Autodesk Fusion 360 part; units mm, degrees
(part 2 of 6)
  spline S37 degree 5 poles (-61.6244, -22.3751) (-61.6253, -22.3767) (-61.6305, -22.3859) (-61.6398, -22.4027) (-61.6532, -22.4272) (-61.6708, -22.4593) (-61.6915, -22.4977) (-61.7119, -22.5363) (-61.7322, -22.5749) (-61.7524, -22.6137) (-61.7724, -22.6527) (-61.7922, -22.6917) (-61.8118, -22.7309) (-61.8313, -22.7703) (-61.8506, -22.8097) (-61.8697, -22.8493) (-61.8887, -22.889) (-61.9075, -22.9288) (-61.9262, -22.9687) (-61.9447, -23.0088) (-61.963, -23.049) (-61.9812, -23.0893) (-61.9993, -23.1297) (-62.0172, -23.1702) (-62.035, -23.2108) (-62.0526, -23.2515) (-62.07, -23.2924) (-62.0873, -23.3333) (-62.1045, -23.3744) (-62.1215, -23.4155) (-62.1384, -23.4568) (-62.1551, -23.4982) (-62.1717, -23.5396) (-62.1882, -23.5812) (-62.2045, -23.6228) (-62.2207, -23.6646) (-62.2367, -23.7064) (-62.2526, -23.7484) (-62.2683, -23.7904) (-62.284, -23.8326) (-62.2995, -23.8748) (-62.3148, -23.9171) (-62.33, -23.9595) (-62.3451, -24.0021) (-62.3601, -24.0446) (-62.3749, -24.0873) (-62.3896, -24.1301) (-62.4012, -24.1644) (-62.4099, -24.1901) (-62.4156, -24.2073) (-62.4185, -24.2159) knots 0.354152 0.354152 0.354152 0.354152 0.354152 0.354152 0.357143 0.371429 0.385714 0.4 0.414286 0.428571 0.442857 0.457143 0.471429 0.485714 0.5 0.514286 0.528571 0.542857 0.557143 0.571429 0.585714 0.6 0.614286 0.628571 0.642857 0.657143 0.671429 0.685714 0.7 0.714286 0.728571 0.742857 0.757143 0.771429 0.785714 0.8 0.814286 0.828571 0.842857 0.857143 0.871429 0.885714 0.9 0.914286 0.928571 0.942857 0.957143 0.971429 0.985714 1 1 1 1 1 1
  arc A19 (-62.4185, -24.2159) -> (-61.8912, -24.6937) centre (-40, 0) ccw
  spline S38 degree 5 poles (-61.8912, -24.6937) (-61.8829, -24.69) (-61.8663, -24.6826) (-61.8416, -24.6714) (-61.8086, -24.6564) (-61.7675, -24.6376) (-61.7265, -24.6187) (-61.6855, -24.5996) (-61.6447, -24.5804) (-61.604, -24.5611) (-61.5634, -24.5416) (-61.5229, -24.5221) (-61.4825, -24.5024) (-61.4422, -24.4825) (-61.402, -24.4626) (-61.362, -24.4425) (-61.322, -24.4223) (-61.2822, -24.402) (-61.2424, -24.3815) (-61.2028, -24.3609) (-61.1633, -24.3402) (-61.1239, -24.3193) (-61.0846, -24.2983) (-61.0454, -24.2772) (-61.0064, -24.256) (-60.9675, -24.2346) (-60.9287, -24.213) (-60.89, -24.1914) (-60.8514, -24.1696) (-60.813, -24.1476) (-60.7747, -24.1255) (-60.7365, -24.1033) (-60.6985, -24.081) (-60.6606, -24.0585) (-60.6228, -24.0358) (-60.5852, -24.013) (-60.5477, -23.9901) (-60.5103, -23.967) (-60.4731, -23.9437) (-60.436, -23.9203) (-60.3991, -23.8968) (-60.3623, -23.8731) (-60.3257, -23.8492) (-60.2892, -23.8252) (-60.2529, -23.801) (-60.2167, -23.7767) (-60.1864, -23.756) (-60.1634, -23.7402) (-60.1476, -23.7293) (-60.1389, -23.7233) (-60.1374, -23.7223) knots -1 -1 -1 -1 -1 -1 -0.985714 -0.971429 -0.957143 -0.942857 -0.928571 -0.914286 -0.9 -0.885714 -0.871429 -0.857143 -0.842857 -0.828571 -0.814286 -0.8 -0.785714 -0.771429 -0.757143 -0.742857 -0.728571 -0.714286 -0.7 -0.685714 -0.671429 -0.657143 -0.642857 -0.628571 -0.614286 -0.6 -0.585714 -0.571429 -0.557143 -0.542857 -0.528571 -0.514286 -0.5 -0.485714 -0.471429 -0.457143 -0.442857 -0.428571 -0.414286 -0.4 -0.385714 -0.371429 -0.357143 -0.354152 -0.354152 -0.354152 -0.354152 -0.354152 -0.354152
  spline S39 degree 3 poles (-59.5346, -23.7468) (-59.5849, -23.7055) (-59.6428, -23.6743) (-59.7672, -23.636) (-59.8326, -23.6291) (-59.9404, -23.6389) (-59.9826, -23.6483) (-60.0636, -23.6778) (-60.102, -23.6977) (-60.1374, -23.7223) knots 0 0 0 0 0.019532 0.019532 0.039064 0.039064 0.051994 0.051994 0.064924 0.064924 0.064924 0.064924
  arc A20 (-59.5346, -23.7468) -> (-59.4691, -23.8006) centre (-40, 0) ccw
  spline S40 degree 3 poles (-59.3272, -24.3869) (-59.3012, -24.3272) (-59.2872, -24.263) (-59.2845, -24.1328) (-59.2958, -24.0681) (-59.3348, -23.9672) (-59.3555, -23.9291) (-59.4061, -23.8593) (-59.4358, -23.8278) (-59.4691, -23.8006) knots 0 0 0 0 0.019532 0.019532 0.039064 0.039064 0.051994 0.051994 0.064924 0.064924 0.064924 0.064924
  spline S41 degree 5 poles (-59.3272, -24.3869) (-59.3279, -24.3886) (-59.3321, -24.3982) (-59.3397, -24.4159) (-59.3507, -24.4416) (-59.365, -24.4753) (-59.3818, -24.5155) (-59.3985, -24.5559) (-59.4149, -24.5964) (-59.4311, -24.6369) (-59.4472, -24.6776) (-59.463, -24.7185) (-59.4787, -24.7594) (-59.4943, -24.8004) (-59.5096, -24.8416) (-59.5248, -24.8829) (-59.5398, -24.9242) (-59.5546, -24.9657) (-59.5693, -25.0073) (-59.5838, -25.049) (-59.5981, -25.0907) (-59.6123, -25.1326) (-59.6263, -25.1746) (-59.6401, -25.2167) (-59.6538, -25.2588) (-59.6673, -25.3011) (-59.6807, -25.3435) (-59.6939, -25.3859) (-59.707, -25.4284) (-59.7199, -25.4711) (-59.7326, -25.5138) (-59.7452, -25.5566) (-59.7577, -25.5995) (-59.77, -25.6424) (-59.7821, -25.6855) (-59.7941, -25.7286) (-59.806, -25.7719) (-59.8177, -25.8152) (-59.8292, -25.8586) (-59.8407, -25.902) (-59.8519, -25.9456) (-59.8631, -25.9892) (-59.874, -26.0329) (-59.8849, -26.0767) (-59.8956, -26.1205) (-59.9062, -26.1645) (-59.9166, -26.2085) (-59.9248, -26.2437) (-59.9309, -26.2702) (-59.935, -26.2879) (-59.937, -26.2967) knots 0.354152 0.354152 0.354152 0.354152 0.354152 0.354152 0.357143 0.371429 0.385714 0.4 0.414286 0.428571 0.442857 0.457143 0.471429 0.485714 0.5 0.514286 0.528571 0.542857 0.557143 0.571429 0.585714 0.6 0.614286 0.628571 0.642857 0.657143 0.671429 0.685714 0.7 0.714286 0.728571 0.742857 0.757143 0.771429 0.785714 0.8 0.814286 0.828571 0.842857 0.857143 0.871429 0.885714 0.9 0.914286 0.928571 0.942857 0.957143 0.971429 0.985714 1 1 1 1 1 1
  arc A21 (-59.937, -26.2967) -> (-59.3653, -26.7205) centre (-40, 0) ccw
  spline S42 degree 5 poles (-59.3653, -26.7205) (-59.3575, -26.716) (-59.3417, -26.707) (-59.3182, -26.6934) (-59.2868, -26.6753) (-59.2477, -26.6525) (-59.2088, -26.6297) (-59.1699, -26.6067) (-59.1312, -26.5836) (-59.0926, -26.5604) (-59.0541, -26.537) (-59.0157, -26.5136) (-58.9774, -26.49) (-58.9393, -26.4664) (-58.9012, -26.4426) (-58.8633, -26.4187) (-58.8255, -26.3946) (-58.7879, -26.3705) (-58.7503, -26.3462) (-58.7129, -26.3219) (-58.6756, -26.2974) (-58.6385, -26.2727) (-58.6014, -26.248) (-58.5645, -26.2231) (-58.5277, -26.1982) (-58.4911, -26.173) (-58.4546, -26.1478) (-58.4182, -26.1225) (-58.382, -26.097) (-58.3459, -26.0714) (-58.31, -26.0457) (-58.2741, -26.0198) (-58.2385, -25.9938) (-58.203, -25.9677) (-58.1676, -25.9414) (-58.1324, -25.9151) (-58.0973, -25.8886) (-58.0624, -25.8619) (-58.0276, -25.8351) (-57.993, -25.8082) (-57.9586, -25.7812) (-57.9243, -25.754) (-57.8902, -25.7266) (-57.8562, -25.6992) (-57.8225, -25.6715) (-57.7888, -25.6438) (-57.7607, -25.6203) (-57.7393, -25.6023) (-57.7247, -25.5898) (-57.7167, -25.583) (-57.7153, -25.5818) knots -1 -1 -1 -1 -1 -1 -0.985714 -0.971429 -0.957143 -0.942857 -0.928571 -0.914286 -0.9 -0.885714 -0.871429 -0.857143 -0.842857 -0.828571 -0.814286 -0.8 -0.785714 -0.771429 -0.757143 -0.742857 -0.728571 -0.714286 -0.7 -0.685714 -0.671429 -0.657143 -0.642857 -0.628571 -0.614286 -0.6 -0.585714 -0.571429 -0.557143 -0.542857 -0.528571 -0.514286 -0.5 -0.485714 -0.471429 -0.457143 -0.442857 -0.428571 -0.414286 -0.4 -0.385714 -0.371429 -0.357143 -0.354152 -0.354152 -0.354152 -0.354152 -0.354152 -0.354152
  spline S43 degree 3 poles (-57.113, -25.5472) (-57.1671, -25.511) (-57.2277, -25.4856) (-57.3553, -25.4597) (-57.421, -25.4593) (-57.5273, -25.4796) (-57.5684, -25.4931) (-57.6462, -25.5303) (-57.6825, -25.5539) (-57.7153, -25.5818) knots 0 0 0 0 0.019532 0.019532 0.039064 0.039064 0.051994 0.051994 0.064924 0.064924 0.064924 0.064924
  arc A22 (-57.113, -25.5472) -> (-57.0425, -25.5943) centre (-40, 0) ccw
  spline S44 degree 3 poles (-56.8438, -26.1639) (-56.8238, -26.1019) (-56.8161, -26.0367) (-56.8262, -25.9068) (-56.8438, -25.8435) (-56.8925, -25.7469) (-56.9168, -25.7111) (-56.974, -25.6466) (-57.0066, -25.6181) (-57.0425, -25.5943) knots 0 0 0 0 0.019532 0.019532 0.039064 0.039064 0.051994 0.051994 0.064924 0.064924 0.064924 0.064924
  spline S45 degree 5 poles (-56.8438, -26.1639) (-56.8443, -26.1656) (-56.8476, -26.1756) (-56.8534, -26.1939) (-56.8619, -26.2206) (-56.8728, -26.2556) (-56.8856, -26.2972) (-56.8981, -26.339) (-56.9105, -26.3809) (-56.9227, -26.4229) (-56.9347, -26.465) (-56.9465, -26.5072) (-56.9581, -26.5494) (-56.9695, -26.5918) (-56.9808, -26.6343) (-56.9918, -26.6768) (-57.0027, -26.7194) (-57.0134, -26.7622) (-57.0239, -26.805) (-57.0342, -26.8479) (-57.0444, -26.8909) (-57.0544, -26.9339) (-57.0642, -26.9771) (-57.0739, -27.0203) (-57.0834, -27.0636) (-57.0927, -27.107) (-57.1018, -27.1505) (-57.1108, -27.194) (-57.1196, -27.2376) (-57.1283, -27.2813) (-57.1368, -27.3251) (-57.1452, -27.3689) (-57.1533, -27.4128) (-57.1614, -27.4568) (-57.1692, -27.5008) (-57.177, -27.5449) (-57.1845, -27.5891) (-57.1919, -27.6333) (-57.1992, -27.6777) (-57.2063, -27.722) (-57.2132, -27.7665) (-57.22, -27.811) (-57.2267, -27.8555) (-57.2332, -27.9002) (-57.2395, -27.9449) (-57.2457, -27.9896) (-57.2518, -28.0344) (-57.2565, -28.0703) (-57.26, -28.0973) (-57.2623, -28.1153) (-57.2634, -28.1243) knots 0.354152 0.354152 0.354152 0.354152 0.354152 0.354152 0.357143 0.371429 0.385714 0.4 0.414286 0.428571 0.442857 0.457143 0.471429 0.485714 0.5 0.514286 0.528571 0.542857 0.557143 0.571429 0.585714 0.6 0.614286 0.628571 0.642857 0.657143 0.671429 0.685714 0.7 0.714286 0.728571 0.742857 0.757143 0.771429 0.785714 0.8 0.814286 0.828571 0.842857 0.857143 0.871429 0.885714 0.9 0.914286 0.928571 0.942857 0.957143 0.971429 0.985714 1 1 1 1 1 1
  arc A23 (-57.2634, -28.1243) -> (-56.653, -28.4899) centre (-40, 0) ccw
  spline S46 degree 5 poles (-56.653, -28.4899) (-56.6456, -28.4847) (-56.6309, -28.4742) (-56.6087, -28.4584) (-56.5793, -28.4373) (-56.5427, -28.4108) (-56.5061, -28.3842) (-56.4697, -28.3575) (-56.4334, -28.3308) (-56.3973, -28.3039) (-56.3612, -28.2769) (-56.3253, -28.2498) (-56.2896, -28.2226) (-56.2539, -28.1953) (-56.2184, -28.1679) (-56.183, -28.1404) (-56.1478, -28.1128) (-56.1126, -28.085) (-56.0777, -28.0572) (-56.0428, -28.0293) (-56.0081, -28.0013) (-55.9735, -27.9731) (-55.9391, -27.9449) (-55.9048, -27.9165) (-55.8707, -27.888) (-55.8367, -27.8595) (-55.8028, -27.8308) (-55.7691, -27.802) (-55.7355, -27.7731) (-55.7021, -27.7441) (-55.6689, -27.7149) (-55.6358, -27.6857) (-55.6028, -27.6563) (-55.57, -27.6269) (-55.5374, -27.5973) (-55.5049, -27.5676) (-55.4726, -27.5377) (-55.4405, -27.5078) (-55.4085, -27.4777) (-55.3767, -27.4476) (-55.3451, -27.4173) (-55.3137, -27.3868) (-55.2824, -27.3563) (-55.2513, -27.3256) (-55.2204, -27.2948) (-55.1897, -27.2639) (-55.164, -27.2377) (-55.1445, -27.2177) (-55.1311, -27.2039) (-55.1238, -27.1964) (-55.1225, -27.1951) knots -1 -1 -1 -1 -1 -1 -0.985714 -0.971429 -0.957143 -0.942857 -0.928571 -0.914286 -0.9 -0.885714 -0.871429 -0.857143 -0.842857 -0.828571 -0.814286 -0.8 -0.785714 -0.771429 -0.757143 -0.742857 -0.728571 -0.714286 -0.7 -0.685714 -0.671429 -0.657143 -0.642857 -0.628571 -0.614286 -0.6 -0.585714 -0.571429 -0.557143 -0.542857 -0.528571 -0.514286 -0.5 -0.485714 -0.471429 -0.457143 -0.442857 -0.428571 -0.414286 -0.4 -0.385714 -0.371429 -0.357143 -0.354152 -0.354152 -0.354152 -0.354152 -0.354152 -0.354152
  spline S47 degree 3 poles (-54.5265, -27.1015) (-54.5839, -27.0708) (-54.6467, -27.0515) (-54.7763, -27.0382) (-54.8417, -27.0442) (-54.9455, -27.0749) (-54.9851, -27.0923) (-55.0588, -27.137) (-55.0926, -27.164) (-55.1225, -27.1951) knots 0 0 0 0 0.019532 0.019532 0.039064 0.039064 0.051994 0.051994 0.064924 0.064924 0.064924 0.064924
  arc A24 (-54.5265, -27.1015) -> (-54.4518, -27.1415) centre (-40, 0) ccw
  spline S48 degree 3 poles (-54.1982, -27.6889) (-54.1843, -27.6253) (-54.1831, -27.5595) (-54.2058, -27.4313) (-54.2296, -27.3701) (-54.2876, -27.2787) (-54.3153, -27.2454) (-54.3785, -27.1868) (-54.4137, -27.1617) (-54.4518, -27.1415) knots 0 0 0 0 0.019532 0.019532 0.039064 0.039064 0.051994 0.051994 0.064924 0.064924 0.064924 0.064924
  spline S49 degree 5 poles (-54.1982, -27.6889) (-54.1985, -27.6907) (-54.2008, -27.7009) (-54.2048, -27.7197) (-54.2106, -27.7471) (-54.2181, -27.783) (-54.2267, -27.8257) (-54.2351, -27.8685) (-54.2433, -27.9114) (-54.2513, -27.9544) (-54.2591, -27.9974) (-54.2667, -28.0406) (-54.2741, -28.0838) (-54.2814, -28.1271) (-54.2884, -28.1704) (-54.2952, -28.2138) (-54.3018, -28.2573) (-54.3083, -28.3009) (-54.3146, -28.3446) (-54.3207, -28.3883) (-54.3266, -28.432) (-54.3323, -28.4759) (-54.3378, -28.5198) (-54.3432, -28.5637) (-54.3484, -28.6078) (-54.3534, -28.6519) (-54.3583, -28.696) (-54.3629, -28.7402) (-54.3675, -28.7845) (-54.3718, -28.8288) (-54.376, -28.8732) (-54.38, -28.9176) (-54.3838, -28.9621) (-54.3875, -29.0067) (-54.391, -29.0513) (-54.3944, -29.0959) (-54.3976, -29.1406) (-54.4006, -29.1854) (-54.4035, -29.2302) (-54.4062, -29.275) (-54.4088, -29.32) (-54.4112, -29.3649) (-54.4134, -29.4099) (-54.4155, -29.455) (-54.4174, -29.5001) (-54.4192, -29.5452) (-54.4209, -29.5904) (-54.4221, -29.6266) (-54.4229, -29.6538) (-54.4234, -29.6719) (-54.4236, -29.6809) knots 0.354152 0.354152 0.354152 0.354152 0.354152 0.354152 0.357143 0.371429 0.385714 0.4 0.414286 0.428571 0.442857 0.457143 0.471429 0.485714 0.5 0.514286 0.528571 0.542857 0.557143 0.571429 0.585714 0.6 0.614286 0.628571 0.642857 0.657143 0.671429 0.685714 0.7 0.714286 0.728571 0.742857 0.757143 0.771429 0.785714 0.8 0.814286 0.828571 0.842857 0.857143 0.871429 0.885714 0.9 0.914286 0.928571 0.942857 0.957143 0.971429 0.985714 1 1 1 1 1 1
  arc A25 (-54.4236, -29.6809) -> (-53.7803, -29.985) centre (-40, 0) ccw
  spline S50 degree 5 poles (-53.7803, -29.985) (-53.7735, -29.9791) (-53.7598, -29.9672) (-53.7393, -29.9493) (-53.7121, -29.9254) (-53.6783, -29.8955) (-53.6445, -29.8654) (-53.6109, -29.8353) (-53.5774, -29.8051) (-53.5441, -29.7748) (-53.5108, -29.7444) (-53.4778, -29.7139) (-53.4448, -29.6833) (-53.412, -29.6527) (-53.3794, -29.6219) (-53.3468, -29.5911) (-53.3145, -29.5601) (-53.2822, -29.5291) (-53.2501, -29.498) (-53.2182, -29.4668) (-53.1864, -29.4355) (-53.1548, -29.4041) (-53.1233, -29.3726) (-53.0919, -29.341) (-53.0607, -29.3093) (-53.0297, -29.2776) (-52.9988, -29.2457) (-52.9681, -29.2138) (-52.9375, -29.1817) (-52.9071, -29.1495) (-52.8769, -29.1173) (-52.8468, -29.0849) (-52.8169, -29.0525) (-52.7872, -29.02) (-52.7576, -28.9873) (-52.7282, -28.9546) (-52.699, -28.9217) (-52.6699, -28.8888) (-52.641, -28.8557) (-52.6124, -28.8226) (-52.5839, -28.7893) (-52.5555, -28.756) (-52.5274, -28.7225) (-52.4995, -28.6889) (-52.4717, -28.6552) (-52.4442, -28.6215) (-52.4212, -28.5929) (-52.4037, -28.5711) (-52.3918, -28.556) (-52.3853, -28.5478) (-52.3841, -28.5464) knots -1 -1 -1 -1 -1 -1 -0.985714 -0.971429 -0.957143 -0.942857 -0.928571 -0.914286 -0.9 -0.885714 -0.871429 -0.857143 -0.842857 -0.828571 -0.814286 -0.8 -0.785714 -0.771429 -0.757143 -0.742857 -0.728571 -0.714286 -0.7 -0.685714 -0.671429 -0.657143 -0.642857 -0.628571 -0.614286 -0.6 -0.585714 -0.571429 -0.557143 -0.542857 -0.528571 -0.514286 -0.5 -0.485714 -0.471429 -0.457143 -0.442857 -0.428571 -0.414286 -0.4 -0.385714 -0.371429 -0.357143 -0.354152 -0.354152 -0.354152 -0.354152 -0.354152 -0.354152
  spline S51 degree 3 poles (-51.8001, -28.3949) (-51.8603, -28.3699) (-51.9247, -28.3569) (-52.0549, -28.3563) (-52.1194, -28.3688) (-52.2197, -28.4094) (-52.2574, -28.4307) (-52.3264, -28.4824) (-52.3574, -28.5126) (-52.3841, -28.5464) knots 0 0 0 0 0.019532 0.019532 0.039064 0.039064 0.051994 0.051994 0.064924 0.064924 0.064924 0.064924
  arc A26 (-51.8001, -28.3949) -> (-51.7219, -28.4273) centre (-40, 0) ccw
  spline S52 degree 3 poles (-51.4158, -28.9472) (-51.4083, -28.8825) (-51.4135, -28.817) (-51.4487, -28.6917) (-51.4784, -28.633) (-51.545, -28.5478) (-51.5758, -28.5174) (-51.6445, -28.4652) (-51.682, -28.4437) (-51.7219, -28.4273) knots 0 0 0 0 0.019532 0.019532 0.039064 0.039064 0.051994 0.051994 0.064924 0.064924 0.064924 0.064924
  spline S53 degree 5 poles (-51.4158, -28.9472) (-51.416, -28.949) (-51.4172, -28.9595) (-51.4194, -28.9786) (-51.4225, -29.0063) (-51.4264, -29.0428) (-51.4308, -29.0862) (-51.435, -29.1296) (-51.4389, -29.1731) (-51.4427, -29.2166) (-51.4462, -29.2603) (-51.4496, -29.3039) (-51.4527, -29.3476) (-51.4557, -29.3914) (-51.4584, -29.4353) (-51.4609, -29.4792) (-51.4633, -29.5231) (-51.4654, -29.5671) (-51.4674, -29.6111) (-51.4692, -29.6552) (-51.4707, -29.6994) (-51.4721, -29.7436) (-51.4734, -29.7878) (-51.4744, -29.8321) (-51.4753, -29.8764) (-51.4759, -29.9208) (-51.4764, -29.9652) (-51.4768, -30.0096) (-51.4769, -30.0541) (-51.4769, -30.0987) (-51.4767, -30.1432) (-51.4763, -30.1879) (-51.4758, -30.2325) (-51.4751, -30.2772) (-51.4742, -30.3219) (-51.4732, -30.3667) (-51.472, -30.4115) (-51.4706, -30.4564) (-51.4691, -30.5012) (-51.4674, -30.5461) (-51.4655, -30.5911) (-51.4635, -30.6361) (-51.4613, -30.6811) (-51.459, -30.7261) (-51.4565, -30.7712) (-51.4539, -30.8163) (-51.4511, -30.8614) (-51.4487, -30.8975) (-51.4469, -30.9247) (-51.4456, -30.9427) (-51.445, -30.9518) knots 0.354152 0.354152 0.354152 0.354152 0.354152 0.354152 0.357143 0.371429 0.385714 0.4 0.414286 0.428571 0.442857 0.457143 0.471429 0.485714 0.5 0.514286 0.528571 0.542857 0.557143 0.571429 0.585714 0.6 0.614286 0.628571 0.642857 0.657143 0.671429 0.685714 0.7 0.714286 0.728571 0.742857 0.757143 0.771429 0.785714 0.8 0.814286 0.828571 0.842857 0.857143 0.871429 0.885714 0.9 0.914286 0.928571 0.942857 0.957143 0.971429 0.985714 1 1 1 1 1 1
  arc A27 (-51.445, -30.9518) -> (-50.7749, -31.1914) centre (-40, 0) ccw
  spline S54 degree 5 poles (-50.7749, -31.1914) (-50.7687, -31.1848) (-50.7563, -31.1716) (-50.7376, -31.1518) (-50.7129, -31.1254) (-50.6821, -31.0922) (-50.6515, -31.059) (-50.621, -31.0257) (-50.5906, -30.9924) (-50.5604, -30.959) (-50.5303, -30.9255) (-50.5004, -30.8919) (-50.4706, -30.8582) (-50.441, -30.8245) (-50.4115, -30.7907) (-50.3821, -30.7568) (-50.353, -30.7229) (-50.3239, -30.6888) (-50.295, -30.6547) (-50.2663, -30.6205) (-50.2377, -30.5862) (-50.2093, -30.5519) (-50.1811, -30.5175) (-50.153, -30.483) (-50.125, -30.4484) (-50.0972, -30.4137) (-50.0696, -30.379) (-50.0422, -30.3442) (-50.0149, -30.3093) (-49.9878, -30.2743) (-49.9609, -30.2392) (-49.9341, -30.2041) (-49.9075, -30.1689) (-49.8811, -30.1336) (-49.8549, -30.0982) (-49.8288, -30.0627) (-49.803, -30.0272) (-49.7773, -29.9915) (-49.7518, -29.9558) (-49.7265, -29.92) (-49.7014, -29.8841) (-49.6765, -29.8482) (-49.6518, -29.8121) (-49.6273, -29.7759) (-49.603, -29.7397) (-49.5789, -29.7034) (-49.5588, -29.6727) (-49.5436, -29.6493) (-49.5331, -29.6331) (-49.5274, -29.6243) (-49.5265, -29.6228) knots -1 -1 -1 -1 -1 -1 -0.985714 -0.971429 -0.957143 -0.942857 -0.928571 -0.914286 -0.9 -0.885714 -0.871429 -0.857143 -0.842857 -0.828571 -0.814286 -0.8 -0.785714 -0.771429 -0.757143 -0.742857 -0.728571 -0.714286 -0.7 -0.685714 -0.671429 -0.657143 -0.642857 -0.628571 -0.614286 -0.6 -0.585714 -0.571429 -0.557143 -0.542857 -0.528571 -0.514286 -0.5 -0.485714 -0.471429 -0.457143 -0.442857 -0.428571 -0.414286 -0.4 -0.385714 -0.371429 -0.357143 -0.354152 -0.354152 -0.354152 -0.354152 -0.354152 -0.354152
  spline S55 degree 3 poles (-48.9601, -29.4148) (-49.0224, -29.3958) (-49.0878, -29.3892) (-49.2174, -29.4014) (-49.2805, -29.4201) (-49.3763, -29.4703) (-49.4117, -29.4952) (-49.4753, -29.5534) (-49.5032, -29.5865) (-49.5265, -29.6228) knots 0 0 0 0 0.019532 0.019532 0.039064 0.039064 0.051994 0.051994 0.064924 0.064924 0.064924 0.064924
  arc A28 (-48.9601, -29.4148) -> (-48.8791, -29.4394) centre (-40, 0) ccw
  spline S56 degree 3 poles (-48.5235, -29.9268) (-48.5224, -29.8617) (-48.534, -29.797) (-48.5813, -29.6757) (-48.6166, -29.6202) (-48.6912, -29.5419) (-48.7249, -29.5147) (-48.7983, -29.4695) (-48.8378, -29.4518) (-48.8791, -29.4394) knots 0 0 0 0 0.019532 0.019532 0.039064 0.039064 0.051994 0.051994 0.064924 0.064924 0.064924 0.064924
  spline S57 degree 5 poles (-48.5235, -29.9268) (-48.5235, -29.9286) (-48.5237, -29.9391) (-48.524, -29.9583) (-48.5244, -29.9863) (-48.5247, -30.0229) (-48.5248, -30.0665) (-48.5247, -30.1101) (-48.5244, -30.1538) (-48.5239, -30.1975) (-48.5231, -30.2413) (-48.5222, -30.2851) (-48.521, -30.3289) (-48.5196, -30.3728) (-48.5181, -30.4166) (-48.5163, -30.4606) (-48.5143, -30.5045) (-48.5121, -30.5485) (-48.5098, -30.5926) (-48.5072, -30.6366) (-48.5045, -30.6807) (-48.5015, -30.7248) (-48.4984, -30.7689) (-48.4951, -30.8131) (-48.4916, -30.8573) (-48.4879, -30.9015) (-48.4841, -30.9458) (-48.48, -30.99) (-48.4758, -31.0343) (-48.4714, -31.0787) (-48.4669, -31.123) (-48.4621, -31.1674) (-48.4572, -31.2118) (-48.4521, -31.2562) (-48.4469, -31.3006) (-48.4415, -31.3451) (-48.4359, -31.3895) (-48.4301, -31.434) (-48.4242, -31.4785) (-48.4181, -31.523) (-48.4119, -31.5676) (-48.4054, -31.6122) (-48.3989, -31.6567) (-48.3921, -31.7013) (-48.3852, -31.7459) (-48.3782, -31.7906) (-48.371, -31.8352) (-48.3651, -31.8709) (-48.3606, -31.8977) (-48.3576, -31.9156) (-48.356, -31.9245) knots 0.354152 0.354152 0.354152 0.354152 0.354152 0.354152 0.357143 0.371429 0.385714 0.4 0.414286 0.428571 0.442857 0.457143 0.471429 0.485714 0.5 0.514286 0.528571 0.542857 0.557143 0.571429 0.585714 0.6 0.614286 0.628571 0.642857 0.657143 0.671429 0.685714 0.7 0.714286 0.728571 0.742857 0.757143 0.771429 0.785714 0.8 0.814286 0.828571 0.842857 0.857143 0.871429 0.885714 0.9 0.914286 0.928571 0.942857 0.957143 0.971429 0.985714 1 1 1 1 1 1
  arc A29 (-48.356, -31.9245) -> (-47.6658, -32.0973) centre (-40, 0) ccw
  spline S58 degree 5 poles (-47.6658, -32.0973) (-47.6602, -32.0901) (-47.6491, -32.0758) (-47.6325, -32.0543) (-47.6105, -32.0255) (-47.5831, -31.9895) (-47.5559, -31.9535) (-47.5288, -31.9174) (-47.5018, -31.8812) (-47.475, -31.845) (-47.4484, -31.8087) (-47.4219, -31.7724) (-47.3956, -31.7359) (-47.3694, -31.6995) (-47.3433, -31.6629) (-47.3175, -31.6263) (-47.2917, -31.5897) (-47.2662, -31.553) (-47.2408, -31.5162) (-47.2155, -31.4793) (-47.1905, -31.4424) (-47.1655, -31.4055) (-47.1408, -31.3684) (-47.1162, -31.3314) (-47.0918, -31.2942) (-47.0676, -31.257) (-47.0435, -31.2197) (-47.0196, -31.1824) (-46.9959, -31.145) (-46.9723, -31.1075) (-46.949, -31.07) (-46.9258, -31.0324) (-46.9028, -30.9947) (-46.8799, -30.957) (-46.8573, -30.9192) (-46.8349, -30.8814) (-46.8126, -30.8434) (-46.7905, -30.8055) (-46.7687, -30.7674) (-46.747, -30.7293) (-46.7255, -30.6911) (-46.7043, -30.6529) (-46.6832, -30.6146) (-46.6624, -30.5762) (-46.6417, -30.5378) (-46.6213, -30.4992) (-46.6043, -30.4668) (-46.5915, -30.442) (-46.5827, -30.4249) (-46.5779, -30.4155) (-46.5771, -30.4139) knots -1 -1 -1 -1 -1 -1 -0.985714 -0.971429 -0.957143 -0.942857 -0.928571 -0.914286 -0.9 -0.885714 -0.871429 -0.857143 -0.842857 -0.828571 -0.814286 -0.8 -0.785714 -0.771429 -0.757143 -0.742857 -0.728571 -0.714286 -0.7 -0.685714 -0.671429 -0.657143 -0.642857 -0.628571 -0.614286 -0.6 -0.585714 -0.571429 -0.557143 -0.542857 -0.528571 -0.514286 -0.5 -0.485714 -0.471429 -0.457143 -0.442857 -0.428571 -0.414286 -0.4 -0.385714 -0.371429 -0.357143 -0.354152 -0.354152 -0.354152 -0.354152 -0.354152 -0.354152
  spline S59 degree 3 poles (-46.0338, -30.1514) (-46.0977, -30.1386) (-46.1634, -30.1384) (-46.2912, -30.1633) (-46.3521, -30.188) (-46.4425, -30.2475) (-46.4753, -30.2757) (-46.5329, -30.3399) (-46.5574, -30.3755) (-46.5771, -30.4139) knots 0 0 0 0 0.019532 0.019532 0.039064 0.039064 0.051994 0.051994 0.064924 0.064924 0.064924 0.064924
  arc A30 (-46.0338, -30.1514) -> (-45.9507, -30.1679) centre (-40, 0) ccw
  spline S60 degree 3 poles (-45.5491, -30.6181) (-45.5544, -30.5532) (-45.5723, -30.49) (-45.6312, -30.3739) (-45.6718, -30.3222) (-45.7538, -30.2515) (-45.7899, -30.2277) (-45.8674, -30.19) (-45.9085, -30.1762) (-45.9507, -30.1679) knots 0 0 0 0 0.019532 0.019532 0.039064 0.039064 0.051994 0.051994 0.064924 0.064924 0.064924 0.064924
  spline S61 degree 5 poles (-45.5491, -30.6181) (-45.549, -30.6199) (-45.5481, -30.6304) (-45.5465, -30.6496) (-45.5442, -30.6774) (-45.5409, -30.7139) (-45.5367, -30.7573) (-45.5323, -30.8007) (-45.5277, -30.8442) (-45.5229, -30.8876) (-45.5179, -30.9311) (-45.5127, -30.9746) (-45.5072, -31.0181) (-45.5015, -31.0616) (-45.4957, -31.1051) (-45.4896, -31.1486) (-45.4833, -31.1922) (-45.4769, -31.2358) (-45.4702, -31.2793) (-45.4633, -31.3229) (-45.4563, -31.3665) (-45.449, -31.4102) (-45.4416, -31.4538) (-45.434, -31.4974) (-45.4262, -31.541) (-45.4182, -31.5847) (-45.41, -31.6283) (-45.4016, -31.672) (-45.3931, -31.7157) (-45.3844, -31.7594) (-45.3755, -31.803) (-45.3664, -31.8467) (-45.3572, -31.8904) (-45.3478, -31.9341) (-45.3382, -31.9778) (-45.3285, -32.0215) (-45.3185, -32.0652) (-45.3084, -32.1089) (-45.2982, -32.1527) (-45.2878, -32.1964) (-45.2772, -32.2401) (-45.2664, -32.2838) (-45.2555, -32.3275) (-45.2444, -32.3713) (-45.2332, -32.415) (-45.2218, -32.4587) (-45.2103, -32.5024) (-45.2009, -32.5374) (-45.1938, -32.5636) (-45.189, -32.5811) (-45.1866, -32.5899) knots 0.354152 0.354152 0.354152 0.354152 0.354152 0.354152 0.357143 0.371429 0.385714 0.4 0.414286 0.428571 0.442857 0.457143 0.471429 0.485714 0.5 0.514286 0.528571 0.542857 0.557143 0.571429 0.585714 0.6 0.614286 0.628571 0.642857 0.657143 0.671429 0.685714 0.7 0.714286 0.728571 0.742857 0.757143 0.771429 0.785714 0.8 0.814286 0.828571 0.842857 0.857143 0.871429 0.885714 0.9 0.914286 0.928571 0.942857 0.957143 0.971429 0.985714 1 1 1 1 1 1
  arc A31 (-45.1866, -32.5899) -> (-44.4828, -32.6941) centre (-40, 0) ccw
  spline S62 degree 5 poles (-44.4828, -32.6941) (-44.4779, -32.6864) (-44.4683, -32.6711) (-44.4539, -32.648) (-44.4348, -32.6173) (-44.4111, -32.5788) (-44.3875, -32.5402) (-44.3641, -32.5016) (-44.3408, -32.463) (-44.3177, -32.4243) (-44.2947, -32.3856) (-44.2719, -32.3468) (-44.2493, -32.308) (-44.2268, -32.2692) (-44.2045, -32.2302) (-44.1823, -32.1913) (-44.1603, -32.1523) (-44.1385, -32.1132) (-44.1168, -32.0741) (-44.0953, -32.035) (-44.0739, -31.9958) (-44.0528, -31.9566) (-44.0318, -31.9173) (-44.0109, -31.878) (-43.9903, -31.8386) (-43.9698, -31.7992) (-43.9495, -31.7598) (-43.9294, -31.7203) (-43.9094, -31.6807) (-43.8897, -31.6411) (-43.8701, -31.6015) (-43.8507, -31.5618) (-43.8315, -31.5221) (-43.8125, -31.4823) (-43.7937, -31.4425) (-43.775, -31.4026) (-43.7566, -31.3627) (-43.7384, -31.3227) (-43.7203, -31.2827) (-43.7025, -31.2427) (-43.6849, -31.2026) (-43.6675, -31.1624) (-43.6503, -31.1222) (-43.6333, -31.082) (-43.6165, -31.0417) (-43.6, -31.0014) (-43.5862, -30.9674) (-43.5759, -30.9414) (-43.5688, -30.9236) (-43.565, -30.9138) (-43.5643, -30.9121) knots -1 -1 -1 -1 -1 -1 -0.985714 -0.971429 -0.957143 -0.942857 -0.928571 -0.914286 -0.9 -0.885714 -0.871429 -0.857143 -0.842857 -0.828571 -0.814286 -0.8 -0.785714 -0.771429 -0.757143 -0.742857 -0.728571 -0.714286 -0.7 -0.685714 -0.671429 -0.657143 -0.642857 -0.628571 -0.614286 -0.6 -0.585714 -0.571429 -0.557143 -0.542857 -0.528571 -0.514286 -0.5 -0.485714 -0.471429 -0.457143 -0.442857 -0.428571 -0.414286 -0.4 -0.385714 -0.371429 -0.357143 -0.354152 -0.354152 -0.354152 -0.354152 -0.354152 -0.354152
  spline S63 degree 3 poles (-43.0494, -30.5976) (-43.1142, -30.5912) (-43.1796, -30.5974) (-43.3044, -30.6347) (-43.3626, -30.6653) (-43.4467, -30.7333) (-43.4766, -30.7646) (-43.5276, -30.8341) (-43.5485, -30.872) (-43.5643, -30.9121) knots 0 0 0 0 0.019532 0.019532 0.039064 0.039064 0.051994 0.051994 0.064924 0.064924 0.064924 0.064924
  arc A32 (-43.0494, -30.5976) -> (-42.9651, -30.6059) centre (-40, 0) ccw
  spline S64 degree 3 poles (-42.5213, -31.0146) (-42.5329, -30.9505) (-42.5569, -30.8893) (-42.627, -30.7796) (-42.6724, -30.7321) (-42.7609, -30.6698) (-42.7992, -30.6497) (-42.88, -30.6197) (-42.9222, -30.6101) (-42.9651, -30.6059) knots 0 0 0 0 0.019532 0.019532 0.039064 0.039064 0.051994 0.051994 0.064924 0.064924 0.064924 0.064924
  spline S65 degree 5 poles (-42.5213, -31.0146) (-42.521, -31.0164) (-42.5191, -31.0267) (-42.5157, -31.0456) (-42.5105, -31.0731) (-42.5037, -31.1091) (-42.4953, -31.1519) (-42.4867, -31.1947) (-42.4779, -31.2374) (-42.4688, -31.2802) (-42.4596, -31.323) (-42.4501, -31.3657) (-42.4404, -31.4085) (-42.4305, -31.4512) (-42.4204, -31.494) (-42.4101, -31.5367) (-42.3996, -31.5795) (-42.3889, -31.6222) (-42.3779, -31.6649) (-42.3668, -31.7076) (-42.3555, -31.7503) (-42.3441, -31.793) (-42.3324, -31.8357) (-42.3205, -31.8784) (-42.3085, -31.921) (-42.2962, -31.9637) (-42.2838, -32.0063) (-42.2712, -32.049) (-42.2585, -32.0916) (-42.2455, -32.1342) (-42.2324, -32.1768) (-42.2191, -32.2194) (-42.2056, -32.262) (-42.192, -32.3045) (-42.1781, -32.3471) (-42.1641, -32.3896) (-42.15, -32.4321) (-42.1357, -32.4746) (-42.1212, -32.5171) (-42.1065, -32.5596) (-42.0917, -32.6021) (-42.0767, -32.6446) (-42.0616, -32.687) (-42.0463, -32.7294) (-42.0308, -32.7718) (-42.0152, -32.8142) (-41.9994, -32.8566) (-41.9866, -32.8905) (-41.977, -32.9159) (-41.9705, -32.9328) (-41.9673, -32.9413) knots 0.354152 0.354152 0.354152 0.354152 0.354152 0.354152 0.357143 0.371429 0.385714 0.4 0.414286 0.428571 0.442857 0.457143 0.471429 0.485714 0.5 0.514286 0.528571 0.542857 0.557143 0.571429 0.585714 0.6 0.614286 0.628571 0.642857 0.657143 0.671429 0.685714 0.7 0.714286 0.728571 0.742857 0.757143 0.771429 0.785714 0.8 0.814286 0.828571 0.842857 0.857143 0.871429 0.885714 0.9 0.914286 0.928571 0.942857 0.957143 0.971429 0.985714 1 1 1 1 1 1
  arc A33 (-41.9673, -32.9413) -> (-41.2566, -32.9761) centre (-40, 0) ccw
  spline S66 degree 5 poles (-41.2566, -32.9761) (-41.2525, -32.968) (-41.2445, -32.9517) (-41.2324, -32.9274) (-41.2164, -32.8949) (-41.1966, -32.8543) (-41.1769, -32.8136) (-41.1573, -32.7729) (-41.138, -32.7322) (-41.1188, -32.6914) (-41.0997, -32.6506) (-41.0808, -32.6098) (-41.0621, -32.5689) (-41.0435, -32.5281) (-41.0251, -32.4872) (-41.0069, -32.4462) (-40.9888, -32.4052) (-40.9709, -32.3642) (-40.9531, -32.3232) (-40.9356, -32.2822) (-40.9182, -32.2411) (-40.901, -32.2) (-40.8839, -32.1588) (-40.867, -32.1176) (-40.8503, -32.0764) (-40.8338, -32.0352) (-40.8175, -31.9939) (-40.8013, -31.9527) (-40.7854, -31.9113) (-40.7696, -31.87) (-40.754, -31.8286) (-40.7386, -31.7872) (-40.7234, -31.7458) (-40.7083, -31.7044) (-40.6935, -31.6629) (-40.6789, -31.6214) (-40.6644, -31.5799) (-40.6502, -31.5383) (-40.6362, -31.4967) (-40.6224, -31.4551) (-40.6088, -31.4135) (-40.5954, -31.3718) (-40.5822, -31.3302) (-40.5692, -31.2885) (-40.5565, -31.2467) (-40.544, -31.205) (-40.5336, -31.1698) (-40.5259, -31.143) (-40.5206, -31.1245) (-40.5177, -31.1144) (-40.5172, -31.1126) knots -1 -1 -1 -1 -1 -1 -0.985714 -0.971429 -0.957143 -0.942857 -0.928571 -0.914286 -0.9 -0.885714 -0.871429 -0.857143 -0.842857 -0.828571 -0.814286 -0.8 -0.785714 -0.771429 -0.757143 -0.742857 -0.728571 -0.714286 -0.7 -0.685714 -0.671429 -0.657143 -0.642857 -0.628571 -0.614286 -0.6 -0.585714 -0.571429 -0.557143 -0.542857 -0.528571 -0.514286 -0.5 -0.485714 -0.471429 -0.457143 -0.442857 -0.428571 -0.414286 -0.4 -0.385714 -0.371429 -0.357143 -0.354152 -0.354152 -0.354152 -0.354152 -0.354152 -0.354152
  spline S67 degree 3 poles (-40.0357, -30.7492) (-40.1008, -30.7491) (-40.1653, -30.7617) (-40.2858, -30.811) (-40.3407, -30.8472) (-40.4178, -30.9231) (-40.4444, -30.9572) (-40.4884, -31.0314) (-40.5054, -31.0712) (-40.5172, -31.1126) knots 0 0 0 0 0.019532 0.019532 0.039064 0.039064 0.051994 0.051994 0.064924 0.064924 0.064924 0.064924
  arc A34 (-40.0357, -30.7492) -> (-39.9509, -30.7492) centre (-40, 0) ccw
  spline S68 degree 3 poles (-39.4692, -31.1124) (-39.487, -31.0498) (-39.5169, -30.9912) (-39.5974, -30.8889) (-39.6473, -30.846) (-39.7414, -30.7928) (-39.7815, -30.7765) (-39.8649, -30.7546) (-39.9078, -30.7491) (-39.9509, -30.7492) knots 0 0 0 0 0.019532 0.019532 0.039064 0.039064 0.051994 0.051994 0.064924 0.064924 0.064924 0.064924
  spline S69 degree 5 poles (-39.4692, -31.1124) (-39.4687, -31.1141) (-39.4658, -31.1242) (-39.4605, -31.1427) (-39.4528, -31.1696) (-39.4424, -31.2047) (-39.4299, -31.2465) (-39.4171, -31.2882) (-39.4041, -31.3299) (-39.3909, -31.3716) (-39.3775, -31.4132) (-39.3639, -31.4549) (-39.3501, -31.4965) (-39.336, -31.538) (-39.3218, -31.5796) (-39.3073, -31.6211) (-39.2927, -31.6626) (-39.2778, -31.7041) (-39.2628, -31.7455) (-39.2476, -31.7869) (-39.2321, -31.8283) (-39.2165, -31.8697) (-39.2007, -31.911) (-39.1847, -31.9523) (-39.1686, -31.9936) (-39.1522, -32.0348) (-39.1357, -32.0761) (-39.1189, -32.1173) (-39.1021, -32.1584) (-39.085, -32.1996) (-39.0678, -32.2407) (-39.0503, -32.2817) (-39.0328, -32.3228) (-39.015, -32.3638) (-38.9971, -32.4048) (-38.979, -32.4458) (-38.9607, -32.4867) (-38.9423, -32.5276) (-38.9237, -32.5685) (-38.905, -32.6093) (-38.8861, -32.6501) (-38.867, -32.6909) (-38.8478, -32.7317) (-38.8284, -32.7724) (-38.8088, -32.8131) (-38.7891, -32.8537) (-38.7692, -32.8944) (-38.7532, -32.9268) (-38.7412, -32.9512) (-38.7331, -32.9674) (-38.729, -32.9755) knots 0.354152 0.354152 0.354152 0.354152 0.354152 0.354152 0.357143 0.371429 0.385714 0.4 0.414286 0.428571 0.442857 0.457143 0.471429 0.485714 0.5 0.514286 0.528571 0.542857 0.557143 0.571429 0.585714 0.6 0.614286 0.628571 0.642857 0.657143 0.671429 0.685714 0.7 0.714286 0.728571 0.742857 0.757143 0.771429 0.785714 0.8 0.814286 0.828571 0.842857 0.857143 0.871429 0.885714 0.9 0.914286 0.928571 0.942857 0.957143 0.971429 0.985714 1 1 1 1 1 1
  arc A35 (-38.729, -32.9755) -> (-38.0183, -32.9404) centre (-40, 0) ccw
  spline S70 degree 5 poles (-38.0183, -32.9404) (-38.0151, -32.932) (-38.0086, -32.915) (-37.999, -32.8896) (-37.9863, -32.8557) (-37.9705, -32.8133) (-37.9549, -32.7709) (-37.9395, -32.7285) (-37.9242, -32.6861) (-37.909, -32.6436) (-37.8941, -32.6012) (-37.8793, -32.5587) (-37.8646, -32.5162) (-37.8502, -32.4737) (-37.8359, -32.4312) (-37.8217, -32.3887) (-37.8078, -32.3461) (-37.794, -32.3036) (-37.7803, -32.261) (-37.7669, -32.2184) (-37.7536, -32.1758) (-37.7405, -32.1332) (-37.7275, -32.0906) (-37.7148, -32.048) (-37.7022, -32.0053) (-37.6898, -31.9627) (-37.6776, -31.92) (-37.6656, -31.8773) (-37.6537, -31.8347) (-37.6421, -31.792) (-37.6306, -31.7493) (-37.6193, -31.7066) (-37.6082, -31.6639) (-37.5973, -31.6211) (-37.5867, -31.5784) (-37.5762, -31.5357) (-37.5659, -31.4929) (-37.5558, -31.4502) (-37.5459, -31.4074) (-37.5362, -31.3647) (-37.5268, -31.3219) (-37.5175, -31.2791) (-37.5085, -31.2364) (-37.4997, -31.1936) (-37.4911, -31.1508) (-37.4827, -31.108) (-37.4759, -31.072) (-37.4708, -31.0445) (-37.4674, -31.0256) (-37.4655, -31.0153) (-37.4652, -31.0135) knots -1 -1 -1 -1 -1 -1 -0.985714 -0.971429 -0.957143 -0.942857 -0.928571 -0.914286 -0.9 -0.885714 -0.871429 -0.857143 -0.842857 -0.828571 -0.814286 -0.8 -0.785714 -0.771429 -0.757143 -0.742857 -0.728571 -0.714286 -0.7 -0.685714 -0.671429 -0.657143 -0.642857 -0.628571 -0.614286 -0.6 -0.585714 -0.571429 -0.557143 -0.542857 -0.528571 -0.514286 -0.5 -0.485714 -0.471429 -0.457143 -0.442857 -0.428571 -0.414286 -0.4 -0.385714 -0.371429 -0.357143 -0.354152 -0.354152 -0.354152 -0.354152 -0.354152 -0.354152
  spline S71 degree 3 poles (-37.0215, -30.6046) (-37.0863, -30.6109) (-37.1493, -30.6298) (-37.2644, -30.6907) (-37.3155, -30.7321) (-37.3847, -30.8152) (-37.4079, -30.8517) (-37.4444, -30.9298) (-37.4575, -30.9711) (-37.4652, -31.0135) knots 0 0 0 0 0.019532 0.019532 0.039064 0.039064 0.051994 0.051994 0.064924 0.064924 0.064924 0.064924
  arc A36 (-37.0215, -30.6046) -> (-36.9372, -30.5963) centre (-40, 0) ccw
  spline S72 degree 3 poles (-36.4222, -30.9105) (-36.4461, -30.85) (-36.4815, -30.7946) (-36.5717, -30.7007) (-36.6255, -30.6629) (-36.7245, -30.6191) (-36.766, -30.6069) (-36.8511, -30.5933) (-36.8943, -30.592) (-36.9372, -30.5963) knots 0 0 0 0 0.019532 0.019532 0.039064 0.039064 0.051994 0.051994 0.064924 0.064924 0.064924 0.064924
  spline S73 degree 5 poles (-36.4222, -30.9105) (-36.4215, -30.9122) (-36.4177, -30.922) (-36.4106, -30.9399) (-36.4002, -30.9658) (-36.3865, -30.9998) (-36.3699, -31.0401) (-36.3531, -31.0804) (-36.3361, -31.1206) (-36.3189, -31.1608) (-36.3015, -31.201) (-36.2839, -31.241) (-36.266, -31.2811) (-36.248, -31.3211) (-36.2297, -31.361) (-36.2113, -31.4009) (-36.1926, -31.4408) (-36.1738, -31.4806) (-36.1547, -31.5204) (-36.1355, -31.5601) (-36.1161, -31.5998) (-36.0965, -31.6394) (-36.0767, -31.679) (-36.0568, -31.7185) (-36.0366, -31.758) (-36.0163, -31.7975) (-35.9958, -31.8369) (-35.9752, -31.8762) (-35.9543, -31.9156) (-35.9333, -31.9548) (-35.9121, -31.994) (-35.8907, -32.0332) (-35.8692, -32.0723) (-35.8475, -32.1114) (-35.8257, -32.1505) (-35.8037, -32.1895) (-35.7815, -32.2284) (-35.7591, -32.2673) (-35.7366, -32.3062) (-35.714, -32.345) (-35.6911, -32.3837) (-35.6682, -32.4224) (-35.645, -32.4611) (-35.6217, -32.4997) (-35.5983, -32.5383) (-35.5747, -32.5768) (-35.551, -32.6153) (-35.5318, -32.6461) (-35.5174, -32.6691) (-35.5078, -32.6845) (-35.503, -32.6922) knots 0.354152 0.354152 0.354152 0.354152 0.354152 0.354152 0.357143 0.371429 0.385714 0.4 0.414286 0.428571 0.442857 0.457143 0.471429 0.485714 0.5 0.514286 0.528571 0.542857 0.557143 0.571429 0.585714 0.6 0.614286 0.628571 0.642857 0.657143 0.671429 0.685714 0.7 0.714286 0.728571 0.742857 0.757143 0.771429 0.785714 0.8 0.814286 0.828571 0.842857 0.857143 0.871429 0.885714 0.9 0.914286 0.928571 0.942857 0.957143 0.971429 0.985714 1 1 1 1 1 1
  arc A37 (-35.503, -32.6922) -> (-34.7991, -32.5876) centre (-40, 0) ccw
  spline S74 degree 5 poles (-34.7991, -32.5876) (-34.7967, -32.5788) (-34.792, -32.5614) (-34.7849, -32.5351) (-34.7755, -32.5001) (-34.764, -32.4564) (-34.7526, -32.4127) (-34.7414, -32.369) (-34.7304, -32.3252) (-34.7195, -32.2815) (-34.7087, -32.2378) (-34.6982, -32.1941) (-34.6878, -32.1503) (-34.6775, -32.1066) (-34.6675, -32.0629) (-34.6576, -32.0192) (-34.6478, -31.9755) (-34.6383, -31.9318) (-34.6289, -31.8881) (-34.6197, -31.8444) (-34.6106, -31.8007) (-34.6017, -31.757) (-34.5931, -31.7133) (-34.5845, -31.6697) (-34.5762, -31.626) (-34.568, -31.5823) (-34.5601, -31.5387) (-34.5523, -31.495) (-34.5447, -31.4514) (-34.5373, -31.4078) (-34.53, -31.3642) (-34.523, -31.3206) (-34.5162, -31.277) (-34.5095, -31.2334) (-34.5031, -31.1898) (-34.4968, -31.1462) (-34.4907, -31.1027) (-34.4849, -31.0592) (-34.4793, -31.0156) (-34.4738, -30.9721) (-34.4686, -30.9287) (-34.4636, -30.8852) (-34.4588, -30.8417) (-34.4542, -30.7983) (-34.4499, -30.7549) (-34.4457, -30.7115) (-34.4425, -30.675) (-34.4401, -30.6471) (-34.4385, -30.628) (-34.4377, -30.6175) (-34.4375, -30.6157) knots -1 -1 -1 -1 -1 -1 -0.985714 -0.971429 -0.957143 -0.942857 -0.928571 -0.914286 -0.9 -0.885714 -0.871429 -0.857143 -0.842857 -0.828571 -0.814286 -0.8 -0.785714 -0.771429 -0.757143 -0.742857 -0.728571 -0.714286 -0.7 -0.685714 -0.671429 -0.657143 -0.642857 -0.628571 -0.614286 -0.6 -0.585714 -0.571429 -0.557143 -0.542857 -0.528571 -0.514286 -0.5 -0.485714 -0.471429 -0.457143 -0.442857 -0.428571 -0.414286 -0.4 -0.385714 -0.371429 -0.357143 -0.354152 -0.354152 -0.354152 -0.354152 -0.354152 -0.354152
  spline S75 degree 3 poles (-34.0361, -30.1653) (-34.1, -30.1779) (-34.1608, -30.2029) (-34.2694, -30.2748) (-34.3161, -30.321) (-34.3769, -30.4105) (-34.3964, -30.4491) (-34.4251, -30.5304) (-34.4341, -30.5727) (-34.4375, -30.6157) knots 0 0 0 0 0.019532 0.019532 0.039064 0.039064 0.051994 0.051994 0.064924 0.064924 0.064924 0.064924
  arc A38 (-34.0361, -30.1653) -> (-33.953, -30.1488) centre (-40, 0) ccw
  spline S76 degree 3 poles (-33.4097, -30.411) (-33.4394, -30.3531) (-33.4801, -30.3015) (-33.579, -30.2168) (-33.6363, -30.1845) (-33.739, -30.1506) (-33.7815, -30.1425) (-33.8676, -30.1373) (-33.9108, -30.1403) (-33.953, -30.1488) knots 0 0 0 0 0.019532 0.019532 0.039064 0.039064 0.051994 0.051994 0.064924 0.064924 0.064924 0.064924
  spline S77 degree 5 poles (-33.4097, -30.411) (-33.4088, -30.4126) (-33.4041, -30.422) (-33.3953, -30.4391) (-33.3824, -30.4639) (-33.3654, -30.4964) (-33.3449, -30.5349) (-33.3243, -30.5733) (-33.3034, -30.6117) (-33.2824, -30.65) (-33.2611, -30.6882) (-33.2396, -30.7264) (-33.2179, -30.7645) (-33.196, -30.8025) (-33.1739, -30.8405) (-33.1517, -30.8784) (-33.1292, -30.9162) (-33.1066, -30.954) (-33.0837, -30.9917) (-33.0607, -31.0293) (-33.0375, -31.0669) (-33.0141, -31.1045) (-32.9905, -31.1419) (-32.9668, -31.1793) (-32.9429, -31.2166) (-32.9188, -31.2539) (-32.8945, -31.2911) (-32.8701, -31.3282) (-32.8455, -31.3653) (-32.8208, -31.4023) (-32.7958, -31.4393) (-32.7707, -31.4762) (-32.7455, -31.513) (-32.7201, -31.5498) (-32.6945, -31.5865) (-32.6687, -31.6231) (-32.6429, -31.6597) (-32.6168, -31.6963) (-32.5906, -31.7327) (-32.5642, -31.7691) (-32.5377, -31.8055) (-32.5111, -31.8417) (-32.4843, -31.8779) (-32.4573, -31.9141) (-32.4302, -31.9502) (-32.4029, -31.9862) (-32.3755, -32.0222) (-32.3535, -32.0509) (-32.3369, -32.0724) (-32.3258, -32.0868) (-32.3202, -32.0939) knots 0.354152 0.354152 0.354152 0.354152 0.354152 0.354152 0.357143 0.371429 0.385714 0.4 0.414286 0.428571 0.442857 0.457143 0.471429 0.485714 0.5 0.514286 0.528571 0.542857 0.557143 0.571429 0.585714 0.6 0.614286 0.628571 0.642857 0.657143 0.671429 0.685714 0.7 0.714286 0.728571 0.742857 0.757143 0.771429 0.785714 0.8 0.814286 0.828571 0.842857 0.857143 0.871429 0.885714 0.9 0.914286 0.928571 0.942857 0.957143 0.971429 0.985714 1 1 1 1 1 1
  arc A39 (-32.3202, -32.0939) -> (-31.63, -31.9209) centre (-40, 0) ccw
  spline S78 degree 5 poles (-31.63, -31.9209) (-31.6285, -31.912) (-31.6255, -31.8941) (-31.621, -31.8673) (-31.6151, -31.8316) (-31.6079, -31.7869) (-31.6009, -31.7423) (-31.594, -31.6977) (-31.5873, -31.6531) (-31.5808, -31.6085) (-31.5744, -31.5639) (-31.5681, -31.5194) (-31.5621, -31.4748) (-31.5562, -31.4303) (-31.5504, -31.3858) (-31.5449, -31.3414) (-31.5395, -31.2969) (-31.5342, -31.2525) (-31.5292, -31.2081) (-31.5243, -31.1637) (-31.5196, -31.1193) (-31.515, -31.075) (-31.5106, -31.0306) (-31.5064, -30.9863) (-31.5024, -30.9421) (-31.4986, -30.8978) (-31.4949, -30.8536) (-31.4915, -30.8094) (-31.4882, -30.7652) (-31.4851, -30.7211) (-31.4822, -30.677) (-31.4794, -30.6329) (-31.4769, -30.5888) (-31.4745, -30.5448) (-31.4724, -30.5008) (-31.4704, -30.4569) (-31.4687, -30.4129) (-31.4671, -30.369) (-31.4658, -30.3252) (-31.4646, -30.2813) (-31.4637, -30.2376) (-31.463, -30.1938) (-31.4625, -30.1501) (-31.4622, -30.1064) (-31.4621, -30.0628) (-31.4622, -30.0192) (-31.4625, -29.9825) (-31.4629, -29.9546) (-31.4632, -29.9354) (-31.4634, -29.9249) (-31.4634, -29.9231) knots -1 -1 -1 -1 -1 -1 -0.985714 -0.971429 -0.957143 -0.942857 -0.928571 -0.914286 -0.9 -0.885714 -0.871429 -0.857143 -0.842857 -0.828571 -0.814286 -0.8 -0.785714 -0.771429 -0.757143 -0.742857 -0.728571 -0.714286 -0.7 -0.685714 -0.671429 -0.657143 -0.642857 -0.628571 -0.614286 -0.6 -0.585714 -0.571429 -0.557143 -0.542857 -0.528571 -0.514286 -0.5 -0.485714 -0.471429 -0.457143 -0.442857 -0.428571 -0.414286 -0.4 -0.385714 -0.371429 -0.357143 -0.354152 -0.354152 -0.354152 -0.354152 -0.354152 -0.354152
  spline S79 degree 3 poles (-31.1081, -29.4355) (-31.1704, -29.4543) (-31.2285, -29.4851) (-31.3295, -29.5673) (-31.3715, -29.6178) (-31.4233, -29.7129) (-31.4389, -29.7532) (-31.4594, -29.837) (-31.4642, -29.88) (-31.4634, -29.9231) knots 0 0 0 0 0.019532 0.019532 0.039064 0.039064 0.051994 0.051994 0.064924 0.064924 0.064924 0.064924
  arc A40 (-31.1081, -29.4355) -> (-31.027, -29.4109) centre (-40, 0) ccw
  spline S80 degree 3 poles (-30.4606, -29.6186) (-30.4958, -29.5639) (-30.5414, -29.5165) (-30.6482, -29.4419) (-30.7083, -29.4154) (-30.8139, -29.3918) (-30.857, -29.3878) (-30.9431, -29.3911) (-30.9858, -29.3983) (-31.027, -29.4109) knots 0 0 0 0 0.019532 0.019532 0.039064 0.039064 0.051994 0.051994 0.064924 0.064924 0.064924 0.064924
  spline S81 degree 5 poles (-30.4606, -29.6186) (-30.4596, -29.6201) (-30.4539, -29.629) (-30.4435, -29.6451) (-30.4283, -29.6685) (-30.4082, -29.6992) (-30.3841, -29.7355) (-30.3597, -29.7717) (-30.3352, -29.8079) (-30.3105, -29.8439) (-30.2856, -29.8799) (-30.2604, -29.9158) (-30.2351, -29.9516) (-30.2096, -29.9873) (-30.1839, -30.0229) (-30.158, -30.0584) (-30.132, -30.0939) (-30.1057, -30.1293) (-30.0793, -30.1646) (-30.0527, -30.1998) (-30.0259, -30.2349) (-29.999, -30.2699) (-29.9719, -30.3049) (-29.9446, -30.3398) (-29.9171, -30.3746) (-29.8895, -30.4093) (-29.8617, -30.444) (-29.8337, -30.4785) (-29.8056, -30.513) (-29.7774, -30.5474) (-29.7489, -30.5818) (-29.7203, -30.616) (-29.6916, -30.6502) (-29.6627, -30.6843) (-29.6336, -30.7183) (-29.6044, -30.7523) (-29.5751, -30.7862) (-29.5456, -30.8199) (-29.5159, -30.8537) (-29.4861, -30.8873) (-29.4562, -30.9209) (-29.4261, -30.9544) (-29.3959, -30.9878) (-29.3655, -31.0211) (-29.335, -31.0544) (-29.3043, -31.0876) (-29.2735, -31.1207) (-29.2488, -31.1471) (-29.2301, -31.1669) (-29.2177, -31.1801) (-29.2115, -31.1867) knots 0.354152 0.354152 0.354152 0.354152 0.354152 0.354152 0.357143 0.371429 0.385714 0.4 0.414286 0.428571 0.442857 0.457143 0.471429 0.485714 0.5 0.514286 0.528571 0.542857 0.557143 0.571429 0.585714 0.6 0.614286 0.628571 0.642857 0.657143 0.671429 0.685714 0.7 0.714286 0.728571 0.742857 0.757143 0.771429 0.785714 0.8 0.814286 0.828571 0.842857 0.857143 0.871429 0.885714 0.9 0.914286 0.928571 0.942857 0.957143 0.971429 0.985714 1 1 1 1 1 1
  arc A41 (-29.2115, -31.1867) -> (-28.5415, -30.9468) centre (-40, 0) ccw
  spline S82 degree 5 poles (-28.5415, -30.9468) (-28.5409, -30.9377) (-28.5397, -30.9197) (-28.5378, -30.8926) (-28.5355, -30.8564) (-28.5327, -30.8113) (-28.5301, -30.7662) (-28.5276, -30.7211) (-28.5253, -30.6761) (-28.5231, -30.6311) (-28.5211, -30.5861) (-28.5193, -30.5411) (-28.5176, -30.4962) (-28.5161, -30.4513) (-28.5148, -30.4065) (-28.5136, -30.3617) (-28.5126, -30.3169) (-28.5117, -30.2722) (-28.511, -30.2275) (-28.5105, -30.1829) (-28.5102, -30.1382) (-28.51, -30.0937) (-28.51, -30.0491) (-28.5102, -30.0046) (-28.5105, -29.9602) (-28.511, -29.9158) (-28.5117, -29.8714) (-28.5126, -29.8271) (-28.5136, -29.7828) (-28.5149, -29.7386) (-28.5163, -29.6944) (-28.5179, -29.6502) (-28.5197, -29.6061) (-28.5217, -29.5621) (-28.5238, -29.5181) (-28.5262, -29.4742) (-28.5288, -29.4303) (-28.5315, -29.3864) (-28.5345, -29.3426) (-28.5376, -29.2989) (-28.541, -29.2553) (-28.5446, -29.2116) (-28.5483, -29.1681) (-28.5523, -29.1246) (-28.5565, -29.0812) (-28.5609, -29.0378) (-28.5649, -29.0013) (-28.568, -28.9736) (-28.5701, -28.9545) (-28.5714, -28.944) (-28.5716, -28.9422) knots -1 -1 -1 -1 -1 -1 -0.985714 -0.971429 -0.957143 -0.942857 -0.928571 -0.914286 -0.9 -0.885714 -0.871429 -0.857143 -0.842857 -0.828571 -0.814286 -0.8 -0.785714 -0.771429 -0.757143 -0.742857 -0.728571 -0.714286 -0.7 -0.685714 -0.671429 -0.657143 -0.642857 -0.628571 -0.614286 -0.6 -0.585714 -0.571429 -0.557143 -0.542857 -0.528571 -0.514286 -0.5 -0.485714 -0.471429 -0.457143 -0.442857 -0.428571 -0.414286 -0.4 -0.385714 -0.371429 -0.357143 -0.354152 -0.354152 -0.354152 -0.354152 -0.354152 -0.354152
  spline S83 degree 3 poles (-28.2657, -28.4222) (-28.3259, -28.447) (-28.3807, -28.4834) (-28.4732, -28.5751) (-28.51, -28.6295) (-28.5522, -28.7291) (-28.5638, -28.7708) (-28.576, -28.8562) (-28.5766, -28.8994) (-28.5716, -28.9422) knots 0 0 0 0 0.019532 0.019532 0.039064 0.039064 0.051994 0.051994 0.064924 0.064924 0.064924 0.064924
  arc A42 (-28.2657, -28.4222) -> (-28.1875, -28.3897) centre (-40, 0) ccw
  spline S84 degree 3 poles (-27.6034, -28.541) (-27.6438, -28.4899) (-27.6938, -28.4473) (-27.8074, -28.3835) (-27.8698, -28.363) (-27.9772, -28.3499) (-28.0205, -28.3502) (-28.1059, -28.3618) (-28.1477, -28.3732) (-28.1875, -28.3897) knots 0 0 0 0 0.019532 0.019532 0.039064 0.039064 0.051994 0.051994 0.064924 0.064924 0.064924 0.064924
  spline S85 degree 5 poles (-27.6034, -28.541) (-27.6023, -28.5424) (-27.5958, -28.5506) (-27.5838, -28.5657) (-27.5663, -28.5875) (-27.5433, -28.616) (-27.5158, -28.6498) (-27.488, -28.6835) (-27.4601, -28.717) (-27.4319, -28.7505) (-27.4036, -28.7838) (-27.3751, -28.8171) (-27.3464, -28.8502) (-27.3175, -28.8832) (-27.2884, -28.9162) (-27.2592, -28.949) (-27.2298, -28.9817) (-27.2002, -29.0144) (-27.1704, -29.0469) (-27.1405, -29.0793) (-27.1104, -29.1117) (-27.0802, -29.1439) (-27.0497, -29.176) (-27.0192, -29.2081) (-26.9884, -29.24) (-26.9575, -29.2719) (-26.9265, -29.3036) (-26.8953, -29.3353) (-26.8639, -29.3669) (-26.8324, -29.3984) (-26.8007, -29.4297) (-26.7689, -29.461) (-26.737, -29.4922) (-26.7049, -29.5233) (-26.6726, -29.5543) (-26.6402, -29.5853) (-26.6077, -29.6161) (-26.575, -29.6468) (-26.5422, -29.6775) (-26.5093, -29.708) (-26.4762, -29.7385) (-26.443, -29.7689) (-26.4096, -29.7992) (-26.3761, -29.8294) (-26.3425, -29.8595) (-26.3087, -29.8895) (-26.2748, -29.9194) (-26.2476, -29.9433) (-26.2271, -29.9612) (-26.2134, -29.9731) (-26.2066, -29.979) knots 0.354152 0.354152 0.354152 0.354152 0.354152 0.354152 0.357143 0.371429 0.385714 0.4 0.414286 0.428571 0.442857 0.457143 0.471429 0.485714 0.5 0.514286 0.528571 0.542857 0.557143 0.571429 0.585714 0.6 0.614286 0.628571 0.642857 0.657143 0.671429 0.685714 0.7 0.714286 0.728571 0.742857 0.757143 0.771429 0.785714 0.8 0.814286 0.828571 0.842857 0.857143 0.871429 0.885714 0.9 0.914286 0.928571 0.942857 0.957143 0.971429 0.985714 1 1 1 1 1 1
  arc A43 (-26.2066, -29.979) -> (-25.5634, -29.6746) centre (-40, 0) ccw